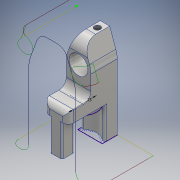
# Autodesk Inventor part: cam-flying-mount
Saved by Autodesk Inventor 2016 (Build 200138000, 138)
## iProperties
Created: 2015-05-15
Part Number: cam-flying-mount
Material: Aluminum 6061
Document SubType Name: Modeling
Designer: as
Mass: 13.9014 g
Surface Area: 42.8978 cm^2
Volume: 5.14867 cm^3
Density: 2.7 g/cm^3
Appearance: Aluminum - Flat
Author: as
Autodesk Inventor part; units mm, degrees
ref_plane "YZ Plane" through (0, 0, 0) normal (1, 0, 0) x (0, 1, 0)
ref_plane "XZ Plane" through (0, 0, 0) normal (0, 1, 0) x (-1, 0, 0)
ref_plane "XY Plane" through (0, 0, 0) normal (0, 0, 1) x (1, 0, 0)
sketch "Sketch1" plane through (0, 0, 0) normal (0, 0, 1) x (1, 0, 0)
  line L0 (-6.5, 4) -> (6.5, 4)
  line L1 (6.5, 4) -> (6.5, -4)
  line L2 (6.5, -4) -> (-6.5, -4)
  line L3 (-6.5, -4) -> (-6.5, 4)
  line L4 (-6.5, 4) -> (6.5, -4) construction
  line L5 (6.5, 4) -> (-6.5, -4) construction
  point P0 (0, 0)
  point P1 (4.5, 1.25)
  point P2 (-4.5, 1.25)
  dimension "d0" = 13
  dimension "d1" = 8
  dimension "d64" = 2.75
  dimension "d65" = 2
  dimension "d66" = 2.75
  dimension "d67" = 2
  constraints: 12 end point, 2 midpoint, 2 parallel, 1 horizontal, 1 perpendicular
  measures "d0" distance of L1.end L2.end
  measures "d1" distance of L0.end L1.end
  measures "d64" distance from line of point (-4.5, 1.25) L0
  measures "d65" distance from line of L3 point (-4.5, 1.25)
  measures "d66" distance from line of L0 point (4.5, 1.25)
  measures "d67" distance from line of point (4.5, 1.25) L1
extrude "Extrusion1" add sketch "Sketch1" along normal blind 48
hole "Hole1" at (-4.5, 1.25, 0) at (4.5, 1.25, 0) direction (0, 0, 1) diameter 2.459 depth 10 tip angle 118 thread size "M3x0.5" class "6H" standard "ISO Metric profile"
sketch "Sketch2" plane through (-6.5, 4, 0) normal (0, 1, 0) x (1, 0, 0)
  line L0 (13, -48) -> (0, -48) projected
  line L1 (0, 0) -> (0, -48) projected
  point P0 (6.5, 0)
  point P1 (6.5, -36)
  dimension "d13" = 12
  dimension "d14" = 6.5
  measures "d13" distance from line of L0 point (6.5, -36)
  measures "d14" distance from line of L1 point (6.5, -36)
hole "Hole2" at (0, 4, 36) direction (0, -1, 0) diameter 10 end through all
hole "Hole3" at (0, 0, 48) direction (0, 0, -1) diameter 3.242 depth 11.8 tip angle 118 thread size "M4x0.7" class "6H" standard "ISO Metric profile"
chamfer "Chamfer1" distance 4 angle 70 2 edges at (-6.5, 0, 48) (6.5, 0, 48) measured on face at (-6, 0, 48) measured on face at (6, 0, 48)
sketch "Sketch3" plane through (-6.3, 4, 0) normal (0, 1, 0) x (1, 0, 0)
  line L0 (6.3, -9.2) -> (6.3, -29.2) construction
  line L1 (1.05, -14.45) -> (1.05, -23.95)
  line L2 (11.55, -23.95) -> (11.55, -14.45)
  arc A0 (1.05, -23.95) -> (11.55, -23.95) centre (6.3, -23.95) ccw
  circle A1 centre (6.3, -36) radius 5.2 projected
  line L3 (6.3, -14.45) -> (6.3, -5.3715) construction
  line L4 (8.7, -7.7715) -> (8.7, -7.7715)
  line L5 (3.9, -7.7715) -> (3.9, -7.7715)
  arc A2 (8.7, -7.7715) -> (3.9, -7.7715) centre (6.3, -7.7715) ccw
  arc A3 (11.55, -14.45) -> (9.9324, -10.6595) centre (6.3, -14.45) ccw
  arc A4 (2.6676, -10.6595) -> (1.05, -14.45) centre (6.3, -14.45) ccw
  arc A5 (8.7, -7.7715) -> (9.9324, -10.6595) centre (12.7, -7.7715) ccw
  arc A6 (2.6676, -10.6595) -> (3.9, -7.7715) centre (-0.1, -7.7715) ccw
  line L6 (12.6, 0) -> (12.6, -36.9748) projected
  point P0 (6.3, 0)
  point P1 (6.3, -19.2)
  point P2 (3.9, -9.7807)
  point P3 (6.3, -9.9107)
  point P4 (8.7, -9.7807)
  point P5 (12.6, -36.8338)
  dimension "d38" = 20
  dimension "d42" = 4
  dimension "d43" = 4
  dimension "d57" = 6.3
  dimension "d58" = 10.5
  dimension "d59" = 6.8
  dimension "d100" = 2.4
  constraints: 17 point on circle, 16 end point, 13 tangent, 6 centre point, 6 point on line, 2 midpoint, 2 parallel, 1 vertical
  measures "d38" distance of L0.start L0.end
  measures "d42" radius of A5
  measures "d43" radius of A6
  measures "d57" distance from line of L6 A0.centre
  measures "d58" distance between parallel lines of L1 L2
  measures "d59" distance of A1.centre L0.end
  measures "d100" radius of A2
extrude "Extrusion2" cut sketch "Sketch3" against normal blind 3.5 contours A4 A6 A2 A5 A3 L2 A0 L1
sketch "Sketch6" plane through (-6.5, -4, 0) normal (0, -1, 0) x (1, 0, 0)
  line L0 (0.2, 0) -> (0, 0) projected
  line L1 (12.8, 0) -> (12.8, 36.9748) projected
  line L2 (0, 0) -> (12.8, 0)
  line L3 (12.8, 0) -> (12.8, 17)
  line L4 (12.8, 17) -> (0, 17)
  line L5 (0, 17) -> (0, 0)
  line L6 (13, 0) -> (13, 37.0101) projected
  line L7 (0, 17) -> (13, 17)
  line L8 (13, 17) -> (13, 23)
  line L9 (13, 23) -> (0, 23)
  line L10 (0, 23) -> (0, 17)
  point P0 (6.5, 0)
  point P1 (12.8, 36.8338)
  point P2 (13, 36.8338)
  dimension "d60" = 17
  dimension "d61" = 6
  constraints: 16 end point, 4 parallel, 2 horizontal, 2 perpendicular, 2 point on line
  measures "d60" distance of L3.end L2.end
  measures "d61" distance of L8.end L7.end
extrude "Extrusion3" add sketch "Sketch6" along normal blind 18 contours L10 L9 L1 L4 | L1 L9 L6 L7
sketch "Sketch12" plane through (-1.7998, -4, 48) normal (0, -1, 0) x (1, 0, 0)
  line L0 (-4.7002, -25) -> (8.2998, -25) projected
  line L1 (8.2998, -25) -> (8.2998, -10.9899) projected
  line L2 (4.2998, 0) -> (8.2998, -10.9899) projected
  line L3 (-0.7002, 0) -> (4.2998, 0) projected
  line L4 (-4.7002, -10.9899) -> (-0.7002, 0) projected
  line L5 (-4.7002, -25) -> (-4.7002, -10.9899) projected
  circle A0 centre (1.7998, -12) radius 5 projected
  point P0 (1.7998, -48)
extrude "Extrusion8" add sketch "Sketch12" along normal blind 6
fillet "Fillet6" radius 4 1 edges at (0, -10, 23)
fillet "Fillet7" radius 6.5 1 edges at (0, -10, 48)
sketch "Sketch7" plane through (6.5, -4, 17) normal (0, 0, -1) x (-1, 0, 0)
  line L0 (13, 8) -> (0, 8) projected
  circle A0 centre (6.5, -4) radius 6
  point P0 (6.5, 4)
  dimension "d68" = 12
  dimension "d69" = 12
  constraints: 1 centre point
  measures "d68" diameter of A0
  measures "d69" distance from line of L0 A0.centre
extrude "Extrusion4" cut sketch "Sketch7" against normal blind 4
sketch "Sketch8" plane through (6.5, -22, 17) normal (0, 0, -1) x (-1, 0, 0)
  circle A0 centre (6.5, 14) radius 6 projected
  circle A1 centre (6.5, 14) radius 7.5
  point P0 (6.5, 22)
  dimension "d72" = 15
  constraints: 1 centre point, 1 coincident
  measures "d72" diameter of A1
extrude "Extrusion5" cut sketch "Sketch8" along normal through all contours A0 | A1
sketch "Sketch9" plane through (0, -8, 21) normal (0, 0, -1) x (-1, 0, 0)
  circle A0 centre (0, 0) radius 5.4
  point P0 (0, 8)
  dimension "d75" = 10.8
  constraints: 1 centre point
  measures "d75" diameter of A0
extrude "Extrusion6" cut sketch "Sketch9" against normal up to surface (2 mm away)
sketch "Sketch10" plane through (6.5, -22, 17) normal (0, 0, -1) x (-1, 0, 0)
  line L0 (3.25, 6.5) -> (3.25, 0)
  line L1 (3.25, 0) -> (9.75, 0)
  line L2 (9.75, 0) -> (9.75, 6.5)
  line L3 (9.75, 6.5) -> (3.25, 6.5)
  line L4 (3.25, 6.5) -> (9.75, 0) construction
  line L5 (3.25, 0) -> (9.75, 6.5) construction
  circle A0 centre (6.5, 14) radius 6 projected
  circle A1 centre (6.5, 14) radius 7.5 projected
  point P0 (6.5, 22)
  point P1 (6.5, 3.25)
  dimension "d78" = 6.5
  dimension "d80" = 6.5
  dimension "d81" = 3.25
  dimension "d95" = 7.5
  constraints: 12 end point, 2 midpoint, 2 parallel, 1 horizontal, 1 perpendicular
  measures "d78" distance of L1.end L0.end
  measures "d80" distance of L1.end L2.end
  measures "d81" distance from line of point (6.5, 22) L2
  measures "d95" distance from line of L3 A1.centre
extrude "Extrusion7" add sketch "Sketch10" along normal up to surface (17 mm away) contours L3 L2 L1 L0
sketch "Sketch11" plane through (3.25, -15.5, 0) normal (0, 0, -1) x (-1, 0, 0)
  line L0 (9.75, 19.5) -> (-3.25, 19.5) projected
  line L1 (-3.25, 19.5) -> (-3.25, 11.5) projected
  line L2 (6.5, 0) -> (0, 0) projected
  point P0 (3.25, 15.5)
  point P1 (3.25, -3.5)
  point P2 (9.55, 19.5)
  point P3 (-3.05, 19.5)
  point P4 (-3.25, 19.3)
  dimension "d85" = 6.5
  dimension "d96" = 3.5
  dimension "d97" = 23
  measures "d85" distance from line of L1 point (3.25, -3.5)
  measures "d96" distance from line of L2 point (3.25, -3.5)
  measures "d97" distance from line of point (3.25, -3.5) L0
hole "Hole5" at (0, -19, 0) direction (0, 0, 1) diameter 2.459 depth 8.8 tip angle 118 thread size "M3x0.5" class "6H" standard "ISO Metric profile"
fillet "Fillet2" radius 1 8 edges at (-6.3443, -4, 8.5) (-6.5, -4, 8.5) (6.3443, -4, 8.5) (6.5, -4, 8.5) (-3.25, -15.5, 8.5) (3.25, -15.5, 8.5) (3.25, -22, 8.5) (-3.25, -22, 8.5)
fillet "Fillet4" radius 3 3 edges at (0, -22, 23) (-6.5, -22, 20) (6.5, -22, 20)
fillet "Fillet5" radius 12 2 edges at (-6.5, -3, 37.0101) (6.5, -3, 37.0101)
sketch "Sketch13" plane through (0, 0, 0) normal (0, 0, -1) x (-1, 0, 0)
  point P0 (4.5, 1.25)
  point P1 (0, -19)
  point P2 (-4.5, 1.25)
equation "\"d66\" = d64"
equation "\"d67\" = d65"
equation "\"d14\" = 0.5 * d0"
equation "\"d23\" = 0.5 * d1"
equation "\"d81\" = 0.5 * d78"
body "Solid1"
